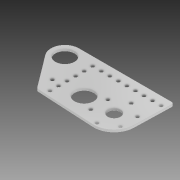
# Autodesk Inventor part: Motor Plate
Saved by Autodesk Inventor 2022 (Build 260153000, 153)
## iProperties
Created: 2022-01-07
Part Number: Motor Plate
Material: Aluminum 6061
Document SubType Name: Modeling
Density: 2.7 g/cm^3
Appearance: Aluminum - Dark
Mass: 31.7871 g
Surface Area: 88.3547 cm^2
Volume: 11.773 cm^3
Mass: 22.6978 g
Surface Area: 68.2049 cm^2
Volume: 8.40659 cm^3
Mass: 86.479 g
Surface Area: 229.336 cm^2
Volume: 32.0293 cm^3
Autodesk Inventor part; units mm, degrees
ref_plane "YZ Plane" through (0, 0, 0) normal (1, 0, 0) x (0, 1, 0)
ref_plane "XZ Plane" through (0, 0, 0) normal (0, 1, 0) x (-1, 0, 0)
ref_plane "XY Plane" through (0, 0, 0) normal (0, 0, 1) x (1, 0, 0)
sketch "CIM" plane through (0, 0, 0) normal (0, 0, 1) x (1, 0, 0)
  circle A0 centre (0, 0) radius 32.004
  circle A1 centre (0, 0) radius 9.525
  circle A2 centre (0, 25.4) radius 2.4892
  circle A3 centre (0, -25.4) radius 2.4892
  dimension "d0" = 64.008
  dimension "d1" = 19.05
  dimension "d2" = 4.9784
  dimension "d5" = 360
  dimension "d7" = 50.8
  measures "d0" diameter of A0
  measures "d1" diameter of A1
  measures "d2" diameter of A2
  measures "d7" distance of A2.centre A3.centre
sketch "VersaKey Patern" plane through (0, 0, 0) normal (0, 0, 1) x (1, 0, 0)
  circle A0 centre (20.6222, 11.9063) radius 2.15
  arc A1 (5.2753, 19.7857) -> (5.9367, 18.5743) centre (6.2412, 19.5268) ccw
  arc A2 (13.1353, 14.4122) -> (14.5161, 14.4442) centre (13.809, 15.1513) ccw
  arc A3 (13.1353, 14.4122) -> (5.9367, 18.5743) centre (0, 0) ccw
  line L0 (5.2753, 19.7857) -> (6.3115, 23.653)
  line L1 (17.347, 17.2752) -> (14.5161, 14.4442)
  arc A4 (7.5745, 24.3491) -> (6.3115, 23.653) centre (7.2774, 23.3942) ccw
  arc A5 (17.3191, 18.7163) -> (7.5745, 24.3491) centre (0, 0) ccw
  arc A6 (17.347, 17.2752) -> (17.3191, 18.7163) centre (16.6399, 17.9823) ccw
  circle A7 centre (-20.6222, 11.9062) radius 2.15
  arc A8 (-14.4973, 14.4613) -> (-13.1175, 14.4285) centre (-13.7902, 15.1684) ccw
  arc A9 (-5.9137, 18.5817) -> (-13.1175, 14.4285) centre (0, 0) ccw
  line L2 (-14.4973, 14.4613) -> (-17.3284, 17.2924)
  arc A10 (-5.9137, 18.5817) -> (-5.251, 19.7934) centre (-6.217, 19.5346) ccw
  arc A11 (-17.2997, 18.7342) -> (-17.3284, 17.2924) centre (-16.6213, 17.9996) ccw
  circle A12 centre (0, 23.8125) radius 2.15
  line L3 (-6.2872, 23.6606) -> (-5.251, 19.7934)
  arc A13 (-7.5492, 24.3569) -> (-17.2997, 18.7342) centre (0, 0) ccw
  arc A14 (-6.2872, 23.6606) -> (-7.5492, 24.3569) centre (-7.2532, 23.4017) ccw
  circle A15 centre (20.6222, -11.9062) radius 2.15
  circle A16 centre (0, -23.8125) radius 2.15
  circle A17 centre (-20.6222, -11.9063) radius 2.15
  arc A18 (-13.1353, -14.4122) -> (-14.5161, -14.4442) centre (-13.809, -15.1513) ccw
  arc A19 (5.9137, -18.5817) -> (5.251, -19.7934) centre (6.217, -19.5346) ccw
  line L4 (6.2872, -23.6606) -> (5.251, -19.7934)
  arc A20 (-13.1353, -14.4122) -> (-5.9367, -18.5743) centre (0, 0) ccw
  arc A21 (-5.2753, -19.7857) -> (-5.9367, -18.5743) centre (-6.2412, -19.5268) ccw
  line L5 (-5.2753, -19.7857) -> (-6.3115, -23.653)
  arc A22 (-7.5745, -24.3491) -> (-6.3115, -23.653) centre (-7.2774, -23.3942) ccw
  arc A23 (-17.347, -17.2752) -> (-17.3191, -18.7163) centre (-16.6399, -17.9823) ccw
  arc A24 (-17.3191, -18.7163) -> (-7.5745, -24.3491) centre (0, 0) ccw
  line L6 (-17.347, -17.2752) -> (-14.5161, -14.4442)
  arc A25 (14.4973, -14.4613) -> (13.1175, -14.4285) centre (13.7902, -15.1684) ccw
  arc A26 (5.9137, -18.5817) -> (13.1175, -14.4285) centre (0, 0) ccw
  line L7 (14.4973, -14.4613) -> (17.3284, -17.2924)
  arc A27 (17.2997, -18.7342) -> (17.3284, -17.2924) centre (16.6213, -17.9996) ccw
  arc A28 (7.5492, -24.3569) -> (17.2997, -18.7342) centre (0, 0) ccw
  arc A29 (6.2872, -23.6606) -> (7.5492, -24.3569) centre (7.2532, -23.4017) ccw
  arc A30 (-19.049, 4.1694) -> (-19.7671, 5.3492) centre (-20.0259, 4.3832) ccw
  arc A31 (-19.049, 4.1694) -> (-19.0542, -4.1458) centre (0, 0) ccw
  arc A32 (-19.7725, -5.3243) -> (-19.0542, -4.1458) centre (-20.0313, -4.3584) ccw
  line L8 (-23.6343, 6.3854) -> (-19.7671, 5.3492)
  arc A33 (-23.6343, 6.3854) -> (-24.8683, 5.6407) centre (-23.8931, 5.4194) ccw
  arc A34 (-24.8683, 5.6407) -> (-24.8742, -5.6148) centre (0, 0) ccw
  line L9 (-19.7725, -5.3243) -> (-23.6399, -6.3606)
  arc A35 (-24.8742, -5.6148) -> (-23.6399, -6.3606) centre (-23.8987, -5.3947) ccw
  arc A36 (19.7725, 5.3243) -> (19.0542, 4.1458) centre (20.0313, 4.3584) ccw
  line L10 (19.7725, 5.3243) -> (23.6399, 6.3606)
  arc A37 (19.049, -4.1694) -> (19.0542, 4.1458) centre (0, 0) ccw
  arc A38 (19.049, -4.1694) -> (19.7671, -5.3492) centre (20.0259, -4.3832) ccw
  line L11 (23.6343, -6.3854) -> (19.7671, -5.3492)
  arc A39 (23.6343, -6.3854) -> (24.8683, -5.6407) centre (23.8931, -5.4194) ccw
  arc A40 (24.8683, -5.6407) -> (24.8742, 5.6148) centre (0, 0) ccw
  arc A41 (24.8742, 5.6148) -> (23.6399, 6.3606) centre (23.8987, 5.3947) ccw
  point P0 (0, 0)
sketch "WCP Gearbox Mounting Pattern" plane through (0, 0, 0) normal (0, 0, 1) x (1, 0, 0)
  circle A0 centre (0, 29.0812) radius 14.2875
  circle A1 centre (-23.8125, 29.0812) radius 2.0193
  circle A2 centre (-57.15, 29.0812) radius 9.525
  circle A3 centre (-57.15, 29.0812) radius 2.4892
  circle A4 centre (23.8125, 29.0812) radius 2.0193
  circle A5 centre (57.15, 29.0812) radius 9.525
  circle A6 centre (57.15, 29.0812) radius 2.4892
  dimension "d43" = 28.575
  dimension "d46" = 360
  dimension "d48" = 19.05
  dimension "d49" = 4.9784
  dimension "d50" = 4.0386
  dimension "d51" = 47.625
  dimension "d52" = 114.3
  measures "d43" diameter of A0
  measures "d48" diameter of A2
  measures "d49" diameter of A3
  measures "d50" diameter of A1
  measures "d51" distance of A4.centre A1.centre
  measures "d52" distance of A5.centre A2.centre
sketch "VersaPlanatery Mounting Pattern" plane through (0, 0, 0) normal (0, 0, 1) x (1, 0, 0)
  line L0 (21.9459, 48.1771) -> (-22.5041, 48.1771)
  line L1 (-22.5041, 48.1771) -> (-22.5041, 3.7271)
  line L2 (-22.5041, 3.7271) -> (21.9459, 3.7271)
  line L3 (21.9459, 3.7271) -> (21.9459, 48.1771)
  line L4 (21.9459, 48.1771) -> (-22.5041, 3.7271) construction
  line L5 (-22.5041, 48.1771) -> (21.9459, 3.7271) construction
  circle A0 centre (-0.2791, 25.9521) radius 14.2875
  circle A1 centre (17.6814, 43.9126) radius 2.4892
  circle A2 centre (-18.2396, 43.9126) radius 2.4892
  circle A3 centre (-18.2396, 7.9916) radius 2.4892
  circle A4 centre (17.6814, 7.9916) radius 2.4892
  point P0 (0.3196, 26.5508)
  dimension "d55" = 44.45
  dimension "d56" = 44.45
  dimension "d57" = 28.575
  dimension "d58" = 4.9784
  dimension "d61" = 360
  dimension "d63" = 50.8
  measures "d55" distance of L2.end L1.end
  measures "d56" distance of L1.end L0.end
  measures "d57" diameter of A0
  measures "d58" diameter of A1
  measures "d63" distance of A4.centre A2.centre
sketch "1.875in Flat Hex Bearing Mount" plane through (0, 0, 0) normal (0, 0, 1) x (1, 0, 0)
  circle A0 centre (-2.1559, 26.2) radius 14.2875
  circle A1 centre (21.6566, 26.2) radius 2.4892
  circle A2 centre (14.6821, 43.0379) radius 2.4892
  circle A3 centre (-18.9938, 43.0379) radius 2.4892
  circle A4 centre (-18.9938, 9.362) radius 2.4892
  circle A5 centre (14.6821, 9.362) radius 2.4892
  circle A6 centre (-25.9684, 26.2) radius 2.4892
  point P0 (-2.1559, 26.2)
  dimension "d66" = 28.575
  dimension "d67" = 4.9784
  dimension "d68" = 4.9784
  dimension "d71" = 360
  dimension "d75" = 360
  dimension "d77" = 47.625
  dimension "d78" = 47.625
  measures "d66" diameter of A0
  measures "d67" diameter of A1
  measures "d68" diameter of A2
  measures "d77" distance of A6.centre A1.centre
  measures "d78" distance of A5.centre A3.centre
sketch "2in Box Tube IsoGrid Pocket Pattern" plane through (0, 0, 0) normal (0, 0, 1) x (1, 0, 0)
  circle A0 centre (-0.1285, 44.8116) radius 2.4892
  line L0 (-6.7243, 60.9984) -> (-2.1082, 53.0031)
  line L1 (1.8513, 53.0031) -> (6.4673, 60.9984)
  line L2 (4.4876, 64.4274) -> (-4.7446, 64.4274)
  line L3 (-25.5285, 70.2116) -> (25.2715, 70.2116) construction
  line L4 (-25.5285, 19.4116) -> (25.2715, 19.4116) construction
  arc A1 (-4.7446, 64.4274) -> (-6.7243, 60.9984) centre (-4.7446, 62.1414) ccw
  arc A2 (6.4673, 60.9984) -> (4.4876, 64.4274) centre (4.4876, 62.1414) ccw
  arc A3 (-2.1082, 53.0031) -> (1.8513, 53.0031) centre (-0.1285, 54.1461) ccw
  line L5 (-17.4446, 47.1928) -> (-8.2124, 47.1928)
  line L6 (-6.2327, 50.6218) -> (-10.8487, 58.6171)
  line L7 (-14.8082, 58.6171) -> (-19.4243, 50.6218)
  arc A4 (-19.4243, 50.6218) -> (-17.4446, 47.1928) centre (-17.4446, 49.4788) ccw
  arc A5 (-10.8487, 58.6171) -> (-14.8082, 58.6171) centre (-12.8285, 57.4741) ccw
  arc A6 (-8.2124, 47.1928) -> (-6.2327, 50.6218) centre (-8.2124, 49.4788) ccw
  line L8 (-10.8487, 31.006) -> (-6.2327, 39.0013)
  line L9 (-8.2124, 42.4303) -> (-17.4446, 42.4303)
  line L10 (-19.4243, 39.0013) -> (-14.8082, 31.006)
  arc A7 (-14.8082, 31.006) -> (-10.8487, 31.006) centre (-12.8285, 32.149) ccw
  arc A8 (-17.4446, 42.4303) -> (-19.4243, 39.0013) centre (-17.4446, 40.1443) ccw
  arc A9 (-6.2327, 39.0013) -> (-8.2124, 42.4303) centre (-8.2124, 40.1443) ccw
  line L11 (6.4673, 28.6248) -> (1.8513, 36.6201)
  line L12 (-2.1082, 36.6201) -> (-6.7243, 28.6248)
  line L13 (-4.7446, 25.1958) -> (4.4876, 25.1958)
  arc A10 (4.4876, 25.1958) -> (6.4673, 28.6248) centre (4.4876, 27.4818) ccw
  arc A11 (-6.7243, 28.6248) -> (-4.7446, 25.1958) centre (-4.7446, 27.4818) ccw
  arc A12 (1.8513, 36.6201) -> (-2.1082, 36.6201) centre (-0.1285, 35.4771) ccw
  line L14 (17.1876, 42.4303) -> (7.9554, 42.4303)
  line L15 (5.9757, 39.0013) -> (10.5918, 31.006)
  line L16 (14.5513, 31.006) -> (19.1673, 39.0013)
  arc A13 (19.1673, 39.0013) -> (17.1876, 42.4303) centre (17.1876, 40.1443) ccw
  arc A14 (10.5918, 31.006) -> (14.5513, 31.006) centre (12.5715, 32.149) ccw
  arc A15 (7.9554, 42.4303) -> (5.9757, 39.0013) centre (7.9554, 40.1443) ccw
  line L17 (10.5918, 58.6171) -> (5.9757, 50.6218)
  line L18 (7.9554, 47.1928) -> (17.1876, 47.1928)
  line L19 (19.1673, 50.6218) -> (14.5513, 58.6171)
  arc A16 (14.5513, 58.6171) -> (10.5918, 58.6171) centre (12.5715, 57.4741) ccw
  arc A17 (17.1876, 47.1928) -> (19.1673, 50.6218) centre (17.1876, 49.4788) ccw
  arc A18 (5.9757, 50.6218) -> (7.9554, 47.1928) centre (7.9554, 49.4788) ccw
  circle A19 centre (12.5715, 63.8616) radius 2.4892
  circle A20 centre (-25.5285, 44.8116) radius 2.4892
  circle A21 centre (25.2715, 44.8116) radius 2.4892
  line L20 (-0.1285, 44.8116) -> (-0.1285, 38.8093) construction
  line L21 (-0.1285, 44.8116) -> (3.6274, 44.8116) construction
  circle A22 centre (-12.8285, 63.8616) radius 2.4892
  circle A23 centre (12.5715, 25.7616) radius 2.4892
  circle A24 centre (-12.8285, 25.7616) radius 2.4892
  dimension "d83" = 4.9784
  dimension "d90" = 50.8
  dimension "d91" = 5.7842
  dimension "d93" = 2.286
  dimension "d96" = 360
  dimension "d98" = 4.7625
  dimension "d99" = 6.35
  dimension "d104" = 25.4
  dimension "d105" = 5.7842
  dimension "d108" = 25.4
  dimension "d115" = 25.4
  dimension "d160" = 8.0839
  dimension "d161" = 8.0839
  measures "d83" diameter of A0
  measures "d90" distance between parallel lines of L3 L4
  measures "d91" distance between parallel lines of L2 L3
  measures "d93" radius of A1
  measures "d98" distance between parallel lines of L17 L1
  measures "d99" distance from line of L3 A19.centre
  measures "d104" distance of A18.centre A4.centre
  measures "d105" distance between parallel lines of L4 L13
  measures "d108" distance of L20.start A20.centre
  measures "d115" distance of L20.start A21.centre
  measures "d160" horizontal distance of A18.centre L20.start
  measures "d161" horizontal distance of A21.centre A17.centre
sketch "2in Box Tube 4 Triangle Pocket Pattern" plane through (0, 0, 0) normal (0, 0, 1) x (1, 0, 0)
  circle A0 centre (-0.7121, 31.493) radius 2.4892
  line L0 (-11.3406, 52.1305) -> (9.9163, 52.1305)
  line L1 (11.5328, 48.228) -> (0.9043, 37.5996)
  line L2 (-2.3286, 37.5996) -> (-12.9571, 48.228)
  arc A1 (-11.3406, 52.1305) -> (-12.9571, 48.228) centre (-11.3406, 49.8445) ccw
  arc A2 (-2.3286, 37.5996) -> (0.9043, 37.5996) centre (-0.7121, 39.216) ccw
  arc A3 (11.5328, 48.228) -> (9.9163, 52.1305) centre (9.9163, 49.8445) ccw
  line L3 (-21.3496, 20.8645) -> (-21.3496, 42.1215)
  line L4 (-17.4472, 43.7379) -> (-6.8187, 33.1094)
  line L5 (-6.8187, 29.8765) -> (-17.4472, 19.2481)
  arc A4 (-21.3496, 20.8645) -> (-17.4472, 19.2481) centre (-19.0636, 20.8645) ccw
  arc A5 (-6.8187, 29.8765) -> (-6.8187, 33.1094) centre (-8.4352, 31.493) ccw
  arc A6 (-17.4472, 43.7379) -> (-21.3496, 42.1215) centre (-19.0636, 42.1215) ccw
  line L6 (9.9163, 10.8555) -> (-11.3406, 10.8555)
  line L7 (-12.9571, 14.7579) -> (-2.3286, 25.3864)
  line L8 (0.9043, 25.3864) -> (11.5328, 14.7579)
  arc A7 (9.9163, 10.8555) -> (11.5328, 14.7579) centre (9.9163, 13.1415) ccw
  arc A8 (0.9043, 25.3864) -> (-2.3286, 25.3864) centre (-0.7121, 23.77) ccw
  arc A9 (-12.9571, 14.7579) -> (-11.3406, 10.8555) centre (-11.3406, 13.1415) ccw
  line L9 (19.9254, 42.1215) -> (19.9254, 20.8645)
  line L10 (16.0229, 19.2481) -> (5.3944, 29.8765)
  line L11 (5.3944, 33.1094) -> (16.0229, 43.7379)
  arc A10 (19.9254, 42.1215) -> (16.0229, 43.7379) centre (17.6394, 42.1215) ccw
  arc A11 (5.3944, 33.1094) -> (5.3944, 29.8765) centre (7.0109, 31.493) ccw
  arc A12 (16.0229, 19.2481) -> (19.9254, 20.8645) centre (17.6394, 20.8645) ccw
  line L12 (-27.744, 56.893) -> (43.6702, 56.893) construction
  line L13 (-27.1477, 6.093) -> (28.101, 6.093) construction
  line L14 (48.5293, 25.3864) -> (59.1578, 14.7579) construction
  arc A13 (48.5293, 25.3864) -> (45.2964, 25.3864) centre (46.9129, 23.77) ccw construction
  line L15 (34.6679, 14.7579) -> (45.2964, 25.3864) construction
  arc A14 (40.8063, 29.8765) -> (40.8063, 33.1094) centre (39.1898, 31.493) ccw construction
  arc A15 (53.0194, 33.1094) -> (53.0194, 29.8765) centre (54.6359, 31.493) ccw construction
  circle A16 centre (46.9129, 31.493) radius 2.4892 construction
  arc A17 (26.2754, 20.8645) -> (30.1778, 19.2481) centre (28.5614, 20.8645) ccw construction
  line L16 (40.8063, 29.8765) -> (30.1778, 19.2481) construction
  line L17 (67.5504, 42.1215) -> (67.5504, 20.8645) construction
  line L18 (26.2754, 20.8645) -> (26.2754, 42.1215) construction
  line L19 (53.0194, 33.1094) -> (63.6479, 43.7379) construction
  line L20 (30.1778, 43.7379) -> (40.8063, 33.1094) construction
  line L21 (45.2964, 37.5996) -> (34.6679, 48.228) construction
  line L22 (36.2844, 52.1305) -> (57.5413, 52.1305) construction
  line L23 (57.5413, 10.8555) -> (36.2844, 10.8555) construction
  arc A18 (36.2844, 52.1305) -> (34.6679, 48.228) centre (36.2844, 49.8445) ccw construction
  line L24 (59.1578, 48.228) -> (48.5293, 37.5996) construction
  arc A19 (59.1578, 48.228) -> (57.5413, 52.1305) centre (57.5413, 49.8445) ccw construction
  arc A20 (45.2964, 37.5996) -> (48.5293, 37.5996) centre (46.9129, 39.216) ccw construction
  line L25 (63.6479, 19.2481) -> (53.0194, 29.8765) construction
  arc A21 (57.5413, 10.8555) -> (59.1578, 14.7579) centre (57.5413, 13.1415) ccw construction
  arc A22 (34.6679, 14.7579) -> (36.2844, 10.8555) centre (36.2844, 13.1415) ccw construction
  arc A23 (30.1778, 43.7379) -> (26.2754, 42.1215) centre (28.5614, 42.1215) ccw construction
  arc A24 (67.5504, 42.1215) -> (63.6479, 43.7379) centre (65.2644, 42.1215) ccw construction
  arc A25 (63.6479, 19.2481) -> (67.5504, 20.8645) centre (65.2644, 20.8645) ccw construction
  circle A26 centre (23.1004, 50.543) radius 2.4892
  circle A27 centre (23.1004, 13.1415) radius 2.4892
  line L26 (23.1004, 50.543) -> (23.1004, 13.1415) construction
  line L27 (-0.7121, 31.493) -> (-0.7121, 20.1913) construction
  circle A28 centre (-24.5246, 50.543) radius 2.4892
  circle A29 centre (-24.5246, 13.1415) radius 2.4892
  dimension "d134" = 4.9784
  dimension "d135" = 2.286
  dimension "d138" = 360
  dimension "d140" = 50.8
  dimension "d141" = 4.7625
  dimension "d142" = 4.7625
  dimension "d143" = 6.35
  dimension "d146" = 47.625
  dimension "d151" = 6.35
  dimension "d162" = 6.35
  measures "d134" diameter of A0
  measures "d135" radius of A1
  measures "d140" distance between parallel lines of L13 L12
  measures "d141" distance between parallel lines of L12 L0
  measures "d142" distance between parallel lines of L13 L6
  measures "d143" distance between parallel lines of L4 L2
  measures "d146" distance of A8.centre A13.centre
  measures "d151" distance between parallel lines of L9 L18
  measures "d162" distance from line of L12 L26.start
sketch "Bag Motor" plane through (0, 0, 0) normal (0, 0, 1) x (1, 0, 0)
  circle A0 centre (-0.9407, 22.0152) radius 20.32
  circle A1 centre (-0.9407, 22.0152) radius 6.0325
  circle A2 centre (-0.9407, 34.5152) radius 2.1
  circle A3 centre (-0.9407, 9.5152) radius 2.1
  point P0 (-0.9407, 22.0152)
  dimension "d165" = 360
  dimension "d167" = 12.065
  dimension "d168" = 25
  dimension "d169" = 4.2
  dimension "d170" = 40.64
  measures "d167" diameter of A1
  measures "d168" distance of A3.centre A2.centre
  measures "d169" diameter of A2
  measures "d170" diameter of A0
sketch "775 Pro" plane through (0, 0, 0) normal (0, 0, 1) x (1, 0, 0)
  arc A0 (-4.434, 16.1665) -> (-14.5364, 8.3491) centre (0, 0) ccw
  arc A1 (-3.376, 12.3089) -> (-11.0678, 6.3569) centre (0, 0) ccw
  arc A2 (-3.376, 12.3089) -> (-4.434, 16.1665) centre (-3.905, 14.2377) ccw
  arc A3 (-14.5364, 8.3491) -> (-11.0678, 6.3569) centre (-12.8021, 7.353) ccw
  arc A4 (14.5364, 8.3491) -> (4.434, 16.1665) centre (0, 0) ccw
  arc A5 (11.0678, 6.3569) -> (3.376, 12.3089) centre (0, 0) ccw
  arc A6 (4.434, 16.1665) -> (3.376, 12.3089) centre (3.905, 14.2377) ccw
  arc A7 (11.0678, 6.3569) -> (14.5364, 8.3491) centre (12.8021, 7.353) ccw
  arc A8 (-11.0678, -6.3569) -> (-3.376, -12.3089) centre (0, 0) ccw
  arc A9 (-4.434, -16.1665) -> (-3.376, -12.3089) centre (-3.905, -14.2377) ccw
  arc A10 (-14.5364, -8.3491) -> (-4.434, -16.1665) centre (0, 0) ccw
  arc A11 (-11.0678, -6.3569) -> (-14.5364, -8.3491) centre (-12.8021, -7.353) ccw
  circle A12 centre (0, 0) radius 8.9535
  circle A13 centre (0, 0) radius 20.6375
  circle A14 centre (14.5, 0) radius 2.0193
  circle A15 centre (-14.5, 0) radius 2.0193
  arc A16 (14.5364, -8.3491) -> (11.0678, -6.3569) centre (12.8021, -7.353) ccw
  arc A17 (4.434, -16.1665) -> (14.5364, -8.3491) centre (0, 0) ccw
  arc A18 (3.376, -12.3089) -> (4.434, -16.1665) centre (3.905, -14.2377) ccw
  arc A19 (3.376, -12.3089) -> (11.0678, -6.3569) centre (0, 0) ccw
  dimension "d173" = 17.907
  dimension "d174" = 41.275
  dimension "d175" = 4.0386
  dimension "d176" = 360
  dimension "d177" = 29
  dimension "d178" = 4
  dimension "d179" = 360
  dimension "d180" = 3.81
  dimension "d181" = 7.81
  dimension "d182" = 360
  measures "d173" diameter of A12
  measures "d174" diameter of A13
  measures "d175" diameter of A14
  measures "d177" distance of A14.centre A15.centre
  measures "d178" radial gap between concentric circles of A0 A1
  measures "d180" radial gap between concentric circles of A5 A12
  measures "d181" distance of A6.centre A2.centre
sketch "Falcon 500" plane through (0, 0, 0) normal (0, 0, 1) x (1, 0, 0)
  circle A0 centre (0, 0) radius 30.1625 construction
  circle A1 centre (0, 0) radius 9.525
  circle A2 centre (0, 25.4) radius 2.4892
  circle A3 centre (0, -25.4) radius 2.4892
  circle A4 centre (21.997, -12.7) radius 2.4892
  circle A5 centre (21.997, 12.7) radius 2.4892
  circle A6 centre (0, 25.4) radius 2.4892
  circle A7 centre (-21.997, 12.7) radius 2.4892
  circle A8 centre (-21.997, -12.7) radius 2.4892
  dimension "d190" = 60.325
  dimension "d191" = 19.05
  dimension "d192" = 4.9784
  dimension "d193" = 360
  dimension "d194" = 50.8
  dimension "d195" = 360
  measures "d190" diameter of A0
  measures "d191" diameter of A1
  measures "d192" diameter of A2
  measures "d194" distance of A2.centre A3.centre
sketch "Standardized T Gusset" plane through (0, 0, 0) normal (0, 0, 1) x (1, 0, 0)
  arc A0 (8.255, 15.5101) -> (16.1511, 6.9174) centre (17.7466, 16.3078) ccw construction
  line L0 (26.2828, 5.196) -> (16.1511, 6.9174) construction
  line L1 (25.4, 0) -> (-25.4, 0) construction
  arc A1 (-1.5954, -9.3904) -> (1.5954, -9.3904) centre (0, 0) ccw construction
  line L2 (26.2828, -5.196) -> (1.5954, -9.3904) construction
  circle A2 centre (25.4, 0) radius 2.4892
  arc A3 (26.2828, -5.196) -> (26.2828, 5.196) centre (25.4, 0) ccw construction
  arc A4 (-16.1511, 6.9174) -> (-8.255, 15.5101) centre (-17.7466, 16.3078) ccw construction
  circle A5 centre (-12.7, 0) radius 2.4892
  line L3 (-1.5954, -9.3904) -> (-26.2828, -5.196) construction
  line L4 (-26.2828, 5.196) -> (-16.1511, 6.9174) construction
  arc A6 (-26.2828, 5.196) -> (-26.2828, -5.196) centre (-25.4, 0) ccw construction
  circle A7 centre (-25.4, 0) radius 2.4892
  circle A8 centre (0, 25.4) radius 2.4892
  line L5 (-8.255, 15.5101) -> (-5.252, 51.2414) construction
  line L6 (0, 0) -> (0, 50.8) construction
  line L7 (8.255, 15.5101) -> (5.252, 51.2414) construction
  circle A9 centre (0, 38.1) radius 2.4892
  circle A10 centre (0, 50.8) radius 2.4892
  arc A11 (5.252, 51.2414) -> (-5.252, 51.2414) centre (0, 50.8) ccw construction
  circle A12 centre (0, 0) radius 2.4892
  circle A13 centre (12.7, 0) radius 2.4892
  point P0 (0, 11.5839)
  dimension "d214" = 4.9784
  dimension "d215" = 25.4
  dimension "d216" = 12.7
  dimension "d217" = 19.05
  dimension "d218" = 10.541
  dimension "d219" = 9.525
  dimension "d220" = 12.7
  dimension "d221" = 25.4
  measures "d214" diameter of A2
  measures "d215" distance of point (0, 0) A8.centre
  measures "d216" distance of A8.centre A9.centre
  measures "d217" diameter of A1
  measures "d218" diameter of A11
  measures "d219" radius of A0
  measures "d220" distance of A2.centre A13.centre
  measures "d221" distance of point (0, 0) A2.centre
sketch "Standardized L Gusset" plane through (0, 0, 0) normal (0, 0, 1) x (1, 0, 0)
  line L0 (0, 0) -> (-25.4, 0) construction
  arc A0 (-16.1511, 6.9174) -> (-8.255, 15.5101) centre (-17.7466, 16.3078) ccw construction
  line L1 (-1.5954, -9.3904) -> (-26.2828, -5.196) construction
  line L2 (-26.2828, 5.196) -> (-16.1511, 6.9174) construction
  arc A1 (-26.2828, 5.196) -> (-26.2828, -5.196) centre (-25.4, 0) ccw construction
  circle A2 centre (0, 25.4) radius 2.4892
  line L3 (-8.255, 15.5101) -> (-5.252, 51.2414) construction
  line L4 (0, 0) -> (0, 50.8) construction
  line L5 (9.4915, 0.7977) -> (5.252, 51.2414) construction
  circle A3 centre (0, 38.1) radius 2.4892
  circle A4 centre (0, 50.8) radius 2.4892
  arc A5 (5.252, 51.2414) -> (-5.252, 51.2414) centre (0, 50.8) ccw construction
  circle A6 centre (-25.4, 0) radius 2.4892
  circle A7 centre (-12.7, 0) radius 2.4892
  circle A8 centre (0, 0) radius 2.4892
  arc A9 (-9.4915, 0.7977) -> (-9.525, 0) centre (0, 0) ccw
  arc A10 (-1.5954, -9.3904) -> (9.4915, 0.7977) centre (0, 0) ccw construction
  point P0 (-7.8691, 13.8492)
  dimension "d260" = 25.4
  dimension "d261" = 12.7
  dimension "d263" = 10.541
  dimension "d273" = 4.9784
  dimension "d276" = 12.7
  dimension "d281" = 9.525
  dimension "d282" = 9.525
  measures "d260" distance of point (0, 0) A2.centre
  measures "d261" distance of A2.centre A3.centre
  measures "d263" diameter of A5
  measures "d273" diameter of A6
  measures "d276" distance of A6.centre A7.centre
  measures "d281" radius of A0
  measures "d282" radius of A10
sketch "Standardized X Gusset" plane through (0, 0, 0) normal (0, 0, 1) x (1, 0, 0)
  arc A0 (8.255, 15.5101) -> (16.1511, 6.9174) centre (17.7466, 16.3078) ccw construction
  line L0 (26.2828, 5.196) -> (16.1511, 6.9174) construction
  circle A1 centre (25.4, 0) radius 2.4892
  arc A2 (26.2828, -5.196) -> (26.2828, 5.196) centre (25.4, 0) ccw construction
  line L1 (25.4, 0) -> (-25.4, 0) construction
  line L2 (26.2828, -5.196) -> (16.1511, -6.9174) construction
  circle A3 centre (0, 0) radius 9.525 construction
  arc A4 (-16.1511, 6.9174) -> (-8.255, 15.5101) centre (-17.7466, 16.3078) ccw construction
  arc A5 (-8.255, -15.5101) -> (-16.1511, -6.9174) centre (-17.7466, -16.3078) ccw construction
  line L3 (-26.2828, 5.196) -> (-16.1511, 6.9174) construction
  circle A6 centre (-25.4, 0) radius 2.4892
  arc A7 (-26.2828, 5.196) -> (-26.2828, -5.196) centre (-25.4, 0) ccw construction
  circle A8 centre (-12.7, 0) radius 2.4892
  circle A9 centre (0, 25.4) radius 2.4892
  line L4 (-8.255, 15.5101) -> (-5.252, 51.2414) construction
  line L5 (8.255, 15.5101) -> (5.252, 51.2414) construction
  line L6 (0, 0) -> (0, 50.8) construction
  circle A10 centre (0, 38.1) radius 2.4892
  circle A11 centre (0, 0) radius 2.4892
  circle A12 centre (0, -25.4) radius 2.4892
  circle A13 centre (12.7, 0) radius 2.4892
  arc A14 (16.1511, -6.9174) -> (8.255, -15.5101) centre (17.7466, -16.3078) ccw construction
  circle A15 centre (0, -38.1) radius 2.4892
  circle A16 centre (0, -50.8) radius 2.4892
  arc A17 (-5.252, -51.2414) -> (5.252, -51.2414) centre (0, -50.8) ccw construction
  line L7 (8.255, -15.5101) -> (5.252, -51.2414) construction
  circle A18 centre (0, 50.8) radius 2.4892
  arc A19 (5.252, 51.2414) -> (-5.252, 51.2414) centre (0, 50.8) ccw construction
  line L8 (-8.255, -15.5101) -> (-5.252, -51.2414) construction
  line L9 (-16.1511, -6.9174) -> (-26.2828, -5.196) construction
  point P0 (0, 1.1165)
  dimension "d314" = 4.9784
  dimension "d315" = 25.4
  dimension "d316" = 12.7
  dimension "d317" = 19.05
  dimension "d318" = 10.541
  dimension "d319" = 9.525
  dimension "d320" = 12.7
  dimension "d321" = 25.4
  dimension "d322" = 12.7
  dimension "d323" = 25.4
  measures "d314" diameter of A1
  measures "d315" distance of point (0, 0) A9.centre
  measures "d316" distance of A9.centre A10.centre
  measures "d317" diameter of A3
  measures "d318" diameter of A19
  measures "d319" radius of A0
  measures "d320" distance of A1.centre A13.centre
  measures "d321" distance of point (0, 0) A1.centre
  measures "d322" distance of A16.centre A15.centre
  measures "d323" distance of A11.centre A12.centre
sketch "Off-set X Gusset" plane through (0, 0, 0) normal (0, 0, 1) x (1, 0, 0)
  line L0 (19.05, 0) -> (-19.05, 0) construction
  line L1 (0, 0) -> (0, 50.8) construction
  circle A0 centre (0, 25.4) radius 2.4892
  circle A1 centre (0, 38.1) radius 2.4892
  circle A2 centre (0, 50.8) radius 2.4892
  arc A3 (5.252, 51.2414) -> (-5.252, 51.2414) centre (0, 50.8) ccw construction
  arc A4 (8.3262, 14.6635) -> (15.6905, 6.1768) centre (17.8177, 15.4612) ccw construction
  line L2 (-8.3262, 14.6635) -> (-5.252, 51.2414) construction
  line L3 (8.3262, 14.6635) -> (5.252, 51.2414) construction
  line L4 (20.2271, 5.1374) -> (15.6905, 6.1768) construction
  circle A5 centre (19.05, 0) radius 2.4892
  arc A6 (20.2271, -5.1374) -> (20.2271, 5.1374) centre (19.05, 0) ccw construction
  line L5 (20.2271, -5.1374) -> (15.6712, -6.1812) construction
  arc A7 (15.6712, -6.1812) -> (8.308, -14.6551) centre (17.7984, -15.4656) ccw construction
  circle A8 centre (0, -24.5934) radius 2.4892
  line L6 (-8.308, -14.6551) -> (-5.2514, -50.442) construction
  line L7 (8.308, -14.6551) -> (5.2514, -50.442) construction
  circle A9 centre (0, 0) radius 9.525 construction
  arc A10 (-20.2271, 5.1374) -> (-20.2271, -5.1374) centre (-19.05, 0) ccw construction
  line L8 (-15.6712, -6.1812) -> (-20.2271, -5.1374) construction
  arc A11 (-15.6905, 6.1768) -> (-8.3262, 14.6635) centre (-17.8177, 15.4612) ccw construction
  circle A12 centre (-6.35, 0) radius 2.4892
  circle A13 centre (6.35, 0) radius 2.4892
  line L9 (-20.2271, 5.1374) -> (-15.6905, 6.1768) construction
  circle A14 centre (-19.05, 0) radius 2.4892
  arc A15 (-8.308, -14.6551) -> (-15.6712, -6.1812) centre (-17.7984, -15.4656) ccw construction
  circle A16 centre (0, -37.2934) radius 2.4892
  circle A17 centre (0, -49.9934) radius 2.4892
  arc A18 (-5.2514, -50.442) -> (5.2514, -50.442) centre (0, -49.9934) ccw construction
  point P0 (0, 1.2591)
  dimension "d364" = 4.9784
  dimension "d365" = 25.4
  dimension "d366" = 12.7
  dimension "d367" = 19.05
  dimension "d368" = 10.541
  dimension "d369" = 9.525
  dimension "d370" = 12.7
  dimension "d371" = 19.05
  dimension "d372" = 12.7
  dimension "d373" = 25.4
  measures "d364" diameter of A5
  measures "d365" distance of point (0, 0) A0.centre
  measures "d366" distance of A0.centre A1.centre
  measures "d367" diameter of A9
  measures "d368" diameter of A3
  measures "d369" radius of A4
  measures "d370" distance of A5.centre A13.centre
  measures "d371" distance of point (0, 0) A5.centre
  measures "d372" distance of A17.centre A16.centre
  measures "d373" distance of A12.centre A8.centre
sketch "Off-set T Gusset" plane through (0, 0, 0) normal (0, 0, 1) x (1, 0, 0)
  circle A0 centre (19.0537, -0.0772) radius 2.4892
  line L0 (0.0037, -0.0772) -> (0.0037, 50.7228) construction
  circle A1 centre (0.0037, 25.3228) radius 2.4892
  circle A2 centre (0.0037, 38.0228) radius 2.4892
  circle A3 centre (0.0037, 50.7228) radius 2.4892
  arc A4 (-2.1236, -9.3616) -> (2.1309, -9.3616) centre (0.0037, -0.0772) ccw construction
  arc A5 (5.2557, 51.1642) -> (-5.2483, 51.1642) centre (0.0037, 50.7228) ccw construction
  arc A6 (-20.2234, 5.0602) -> (-20.2234, -5.2145) centre (-19.0463, -0.0772) ccw construction
  arc A7 (20.2308, -5.2145) -> (20.2308, 5.0602) centre (19.0537, -0.0772) ccw construction
  line L1 (20.2308, -5.2145) -> (2.1309, -9.3616) construction
  line L2 (-2.1236, -9.3616) -> (-20.2234, -5.2145) construction
  line L3 (20.2308, 5.0602) -> (15.6942, 6.0996) construction
  line L4 (-20.2234, 5.0602) -> (-15.6868, 6.0996) construction
  line L5 (8.3299, 14.5863) -> (5.2557, 51.1642) construction
  line L6 (-8.3225, 14.5863) -> (-5.2483, 51.1642) construction
  arc A8 (8.3299, 14.5863) -> (15.6942, 6.0996) centre (17.8214, 15.3841) ccw construction
  arc A9 (-15.6868, 6.0996) -> (-8.3225, 14.5863) centre (-17.814, 15.3841) ccw construction
  line L7 (19.0537, -0.0772) -> (-19.0463, -0.0772) construction
  circle A10 centre (6.3537, -0.0772) radius 2.4892
  circle A11 centre (-6.3463, -0.0772) radius 2.4892
  circle A12 centre (-19.0463, -0.0772) radius 2.4892
  point P0 (0, 11.5839)
  dimension "d398" = 4.9784
  dimension "d399" = 25.4
  dimension "d400" = 12.7
  dimension "d401" = 19.05
  dimension "d402" = 10.541
  dimension "d403" = 9.525
  dimension "d405" = 19.05
  dimension "d417" = 12.7
  measures "d398" diameter of A0
  measures "d399" distance of point (0.004, -0.077) A1.centre
  measures "d400" distance of A1.centre A2.centre
  measures "d401" diameter of A4
  measures "d402" diameter of A5
  measures "d403" radius of A8
  measures "d405" distance of point (0.004, -0.077) A0.centre
  measures "d417" distance of A0.centre A10.centre
sketch "Retained Bearing" plane through (0, 0, 0) normal (0, 0, 1) x (1, 0, 0)
  circle A0 centre (-51.0531, -16.1798) radius 14.2875
  circle A1 centre (-51.0531, -34.5948) radius 2.4892 construction
  circle A2 centre (-51.0531, -34.5948) radius 6.35 construction
  circle A3 centre (-35.1052, -6.9723) radius 2.4892 construction
  circle A4 centre (-35.1052, -6.9723) radius 6.35 construction
  circle A5 centre (-67.0009, -6.9723) radius 2.4892 construction
  circle A6 centre (-67.0009, -6.9723) radius 6.35 construction
  point P0 (-5.1155, 13.4934)
  dimension "d422" = 28.575
  dimension "d423" = 4.9784
  dimension "d424" = 12.7
  dimension "d426" = 18.415
  dimension "d429" = 360
  measures "d422" diameter of A0
  measures "d423" diameter of A1
  measures "d424" diameter of A2
  measures "d426" distance of point (-51.053, -16.18) A1.centre
sketch "Sketch21" plane through (0, 0, 0) normal (0, 1, 0) x (-1, 0, 0)
  circle A0 centre (0, 0) radius 2.4892
  line L0 (-1.1084, 0) -> (0, 0) construction
  line L1 (0, 0) -> (0, 1.1837) construction
  circle A1 centre (-12.7, 0) radius 2.4892
  circle A2 centre (-25.4, 0) radius 2.4892
  circle A3 centre (-38.1, 0) radius 2.4892
  circle A4 centre (-50.8, 0) radius 2.4892
  circle A5 centre (-63.5, 0) radius 2.4892
  circle A6 centre (0, 12.7) radius 2.4892
  circle A7 centre (0, 25.4) radius 2.4892
  circle A8 centre (0, 38.1) radius 2.4892
  circle A9 centre (0, 50.8) radius 2.4892
  circle A10 centre (0, 63.5) radius 2.4892
  circle A11 centre (-31.75, 44.45) radius 14.2875
  circle A12 centre (33.3375, 7.9375) radius 14.2875
  arc A13 (33.3375, -12.7) -> (49.8475, 20.32) centre (33.3375, 7.9375) ccw
  circle A14 centre (-76.2762, 44.45) radius 6.3881 construction
  circle A15 centre (-31.75, 44.45) radius 38.1381 construction
  circle A16 centre (-31.75, 44.45) radius 22.2339 construction
  line L2 (-107.95, -12.7) -> (33.3375, -12.7)
  line L3 (49.8475, 20.32) -> (12.7, 69.85)
  line L4 (-12.7, 65.1668) -> (-12.7, 12.7) construction
  line L5 (-12.7, 12.7) -> (-37.3935, 12.7) construction
  line L6 (-76.2762, 69.85) -> (-76.2762, 19.05) construction
  line L7 (12.7, 69.85) -> (-74.6492, 74.5686)
  line L8 (-107.95, -12.7) -> (-106.4283, 45.2419)
  arc A17 (-74.6492, 74.5686) -> (-106.4283, 45.2419) centre (-76.2762, 44.45) ccw
  circle A18 centre (-76.2, 0) radius 2.4892
  circle A19 centre (-88.9, 0) radius 2.4892
  circle A20 centre (-101.6, 0) radius 2.4892
  circle A21 centre (12.6454, 47.3206) radius 2.4892
  line L9 (-31.75, 44.45) -> (12.6454, 47.3206) construction
  line L10 (12.6454, 47.3206) -> (33.3375, 7.9375) construction
  circle A22 centre (12.6454, 47.3206) radius 6.35 construction
  circle A23 centre (-76.2762, 44.45) radius 30.1625 construction
  circle A24 centre (-76.2762, 44.45) radius 9.525
  circle A25 centre (-76.2762, 69.85) radius 2.4892
  circle A26 centre (-76.2762, 19.05) radius 2.4892
  circle A27 centre (-54.2792, 31.75) radius 2.4892
  circle A28 centre (-54.2792, 57.15) radius 2.4892
  circle A29 centre (-76.2762, 69.85) radius 2.4892
  circle A30 centre (-98.2732, 57.15) radius 2.4892
  circle A31 centre (-98.2732, 31.75) radius 2.4892
  dimension "d433" = 4.9784
  dimension "d436" = 12.7
  dimension "d443" = 12.7
  dimension "d448" = 28.575
  dimension "d449" = 6.35
  dimension "d451" = 12.7762
  dimension "d452" = 76.2762
  dimension "d453" = 44.4679
  dimension "d454" = 12.7
  dimension "d455" = 33.3375
  dimension "d456" = 12.7
  dimension "d457" = 6.35
  dimension "d458" = 12.7
  dimension "d459" = 12.7
  dimension "d460" = 31.75
  dimension "d461" = 19.05
  dimension "d466" = 6.35
  dimension "d467" = 4.9784
  dimension "d468" = 12.7
  constraints: 23 centre point, 22 end point, 5 coincident, 4 point on circle, 4 tangent, 3 horizontal, 3 vertical, 2 perpendicular, 1 equal length, 1 equal radius, 34 other
  measures "d433" diameter of A0
  measures "d436" distance of L0.end A1.centre
  measures "d443" distance of L0.end A6.centre
  measures "d448" diameter of A11
  measures "d449" radial gap between concentric circles of A12 A13
  measures "d451" diameter of A14
  measures "d452" diameter of A15
  measures "d453" diameter of A16
  measures "d454" distance from line of L2 point (0, 0)
  measures "d455" horizontal distance of point (0, 0) L10.end
  measures "d456" horizontal distance of L3.end A10.centre
  measures "d457" vertical distance of L3.end A10.centre
  measures "d458" distance from line of point (0, 0) L5
  measures "d459" distance from line of L4 point (0, 0)
  measures "d460" distance from line of L5 A11.centre
  measures "d461" distance from line of L4 A11.centre
  measures "d466" horizontal distance of L2.start A20.centre
  measures "d467" diameter of A21
  measures "d468" diameter of A22
extrude "Extrusion1" add sketch "Sketch21" along normal blind 3.175
fillet "Fillet1" radius 3.175 2 edges at (-12.7, 1.5875, 69.85) (107.95, 1.5875, -12.7)
equation "\"d105\" = d91"
equation "\"d142\" = d141"
body "Solid1"
